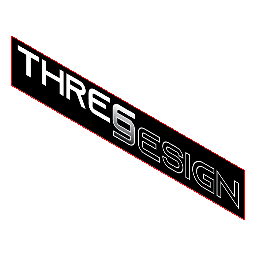
BF15 Endstop Mod (Autodesk Fusion 360 archive; units mm, degrees)
design "Base Parameters"
Autodesk Fusion 360 part; units mm, degrees
sketch "Steel Profile" plane through (0, 0, 0) normal (0, 1, 0) x (1, 0, 0)
  line L0 (-25.05, -37.55) -> (25.05, -37.55)
  line L1 (25.05, -37.55) -> (25.05, 37.55)
  line L2 (25.05, 37.55) -> (-25.05, 37.55)
  line L3 (-25.05, 37.55) -> (-25.05, -37.55)
  line L4 (-25.05, 0) -> (25.05, 0) construction
  dimension "d32" = 75.1
  dimension "d33" = 50.1
  constraint horizontal L0
  constraint vertical L1
  constraint horizontal L2
  constraint vertical L3
  constraint midpoint L3 L4.start
  constraint midpoint L1 L4.end
  constraint midpoint origin L4
  measures "d32" distance of L0.start L2.end
  measures "d33" distance of L0.start L0.end
extrude "Extrude1" add sketch "Steel Profile" along normal blind 100
shell "Shell1" thickness 3.2 removed faces 2 at (-8.35, 100, -12.5167) at (-8.35, 0, -12.5167)
fillet "Fillet1" radius 4 8 edges at (-21.85, 50, 34.35) (-25.05, 50, 37.55) (25.05, 50, 37.55) (21.85, 50, 34.35) (21.85, 50, -34.35) (25.05, 50, -37.55) (-25.05, 50, -37.55) (-21.85, 50, -34.35)
equation "frameX = 1650 mm"
equation "frameY = 1500 mm"
equation "steelWide = 75.1 mm"
equation "steelNarrow = 50.1 mm"
equation "steelThick = 3.2 mm"
equation "steelRadius = 4 mm"
equation "d32 = steelWide"
equation "d33 = steelNarrow"
equation "d36 = steelThick"
equation "d37 = steelRadius"
equation "wasteThick = 10 mm"
equation "optionalXGantryTall = steelWide"
equation "optionalXGantryNarrow = steelNarrow"
equation "angleLong = 75 mm"
equation "angleShort = 50 mm"
equation "angleThick = 6 mm"
equation "angleRadius = 0.1 mm"
equation "yRailHoles = floor(( frameY - 200 mm ) / 60)"
equation "facePlateThickness = 10 mm"
equation "optionalYRailLong = steelWide"
equation "optionalYRailShort = steelNarrow"
equation "xBallScrewDiameter = 16 mm"
equation "yBallScrewDiameter = 16 mm"
named bodies: "Steel Section - 100mm"
